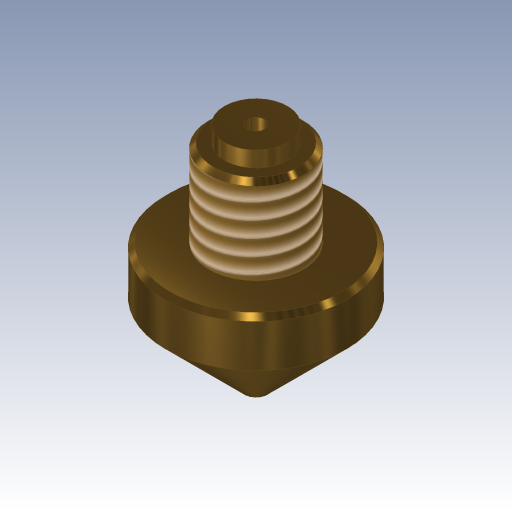
# Autodesk Inventor part: BT003_huenin20_23
Saved by Autodesk Inventor 2023.3 (Build 273359000, 359)
## iProperties
Company: HTBLA Kaindorf
RuleStatus: InUse
Created: 2023-08-12
Part Number: BT003_huenin20_23
Project: Fiberprinter-Hotend
Material: Messing
Description: Nozzel_extender
Document SubType Name: Modeling
Designer: huenin20
Density: 8.49 g/cm^3
Appearance: Messing - poliert
Mass: 5.62144 g
Surface Area: 5.12966 cm^2
Volume: 0.662125 cm^3
AfterDocNew0: iProperties-Editor_aufrufen
Author: nicob
Keywords: 2023
Autodesk Inventor part; units mm, degrees
ref_plane "YZ Plane" through (0, 0, 0) normal (1, 0, 0) x (0, 1, 0)
ref_plane "XZ Plane" through (0, 0, 0) normal (0, 1, 0) x (-1, 0, 0)
ref_plane "XY Plane" through (0, 0, 0) normal (0, 0, 1) x (1, 0, 0)
sketch "Skizze3" plane through (0, 0, 0) normal (1, 0, 0) x (0, 1, 0)
  line L0 (0, 0) -> (0, 30.5982)
  line L1 (0, 0) -> (-0.75, 0)
  line L2 (-0.75, 0) -> (-5.75, 5)
  line L3 (-5.75, 5) -> (-5.75, 8)
  line L4 (-5.75, 8) -> (-3, 8)
  line L5 (-3, 8) -> (-3, 13.5)
  line L6 (-3, 13.5) -> (-2, 13.5)
  line L7 (-2, 13.5) -> (-2, 14.5)
  line L8 (-2, 14.5) -> (-0.55, 14.5)
  line L9 (-0.55, 14.5) -> (-0.55, 0)
  point P0 (-2.5, 13.5)
  dimension "d7" = 1.5
  dimension "d9" = 11.5
  dimension "d11" = 6
  dimension "d12" = 4
  dimension "d13" = 1
  dimension "d15" = 1.1
  dimension "d37" = 45
  dimension "d38" = 3
  dimension "d39" = 6.5
  constraints: 20 end point, 6 perpendicular, 2 horizontal, 1 midpoint, 1 point on line, 1 vertical
  measures "d7" diameter of L1.end L0
  measures "d9" diameter of L3 L0
  measures "d11" diameter of L5 L0
  measures "d12" diameter of L7 L0
  measures "d13" distance from line of point (-2.5, 13.5) L8
  measures "d15" diameter of L9 L0
  measures "d37" angle of L3 L2
  measures "d38" distance of L2.end L3.end
  measures "d39" distance between parallel lines of L8 L4
revolve "Umdrehung1" add sketch "Skizze3" angle 360 about axis through (0, 0, 0) along (0, 0, 1)
thread "Gewinde1" size "M6x1" class "6g" standard "ISO Metric profile" length 15
chamfer "Fase1" distance 0.3 angle 45 2 edges at (0, 3, 13.5) (0, 5.75, 8)
